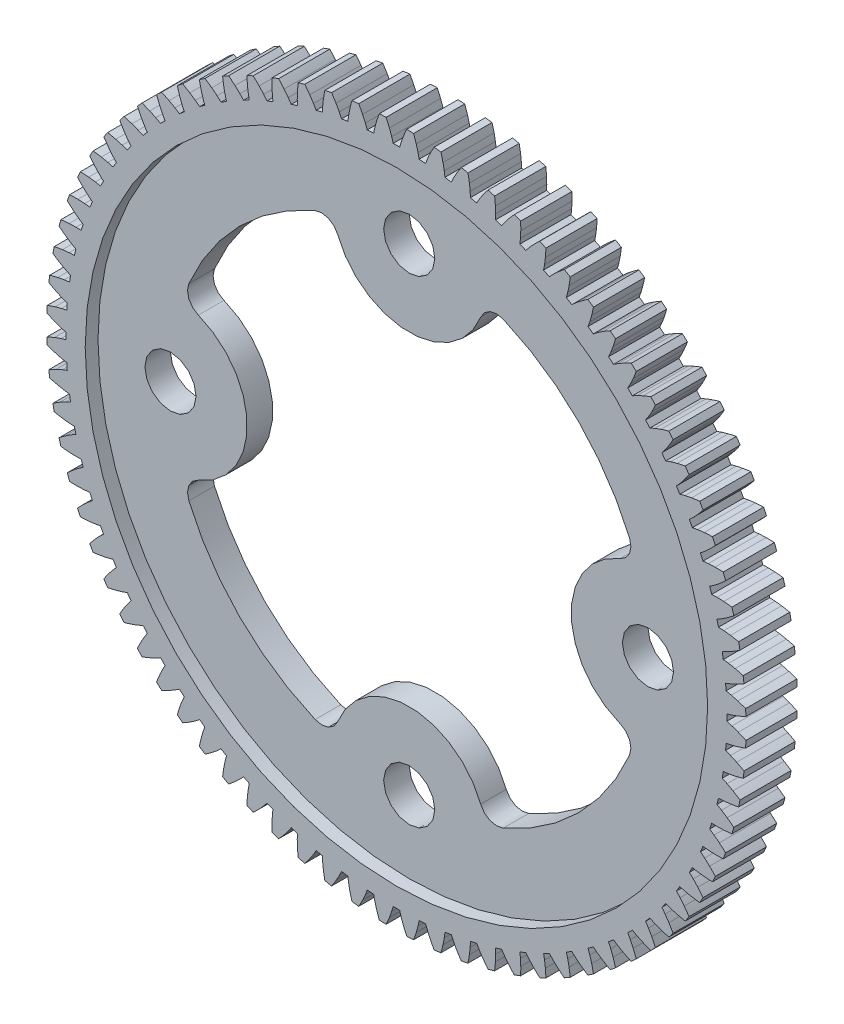
# Autodesk Inventor part: 歯車m0.5.z80
Saved by Autodesk Inventor 2020 (Build 240168000, 168)
## iProperties
Part Number: 歯車m0.5.z80
Material: 鋼、高強度、低合金
Document SubType Name: Modeling
Designer: 雪村
Density: 7.85 g/cm^3
Appearance: 鋼 - つや出し
Mass: 10.9737 g
Surface Area: 25.8897 cm^2
Volume: 1.39793 cm^3
Author: 雪村
Autodesk Inventor part; units mm, degrees
(part 1 of 4)
ref_plane "YZ Plane" through (0, 0, 0) normal (1, 0, 0) x (0, 1, 0)
ref_plane "XZ Plane" through (0, 0, 0) normal (0, 1, 0) x (-1, 0, 0)
ref_plane "XY Plane" through (0, 0, 0) normal (0, 0, 1) x (1, 0, 0)
sketch "スケッチ1" plane through (0, 0, 0) normal (0, 0, 1) x (1, 0, 0)
  arc A0 (1.2215, 23.1029) -> (1.1332, 22.8025) centre (6.2327, 21.4655) ccw
  arc A1 (1.3553, 23.4735) -> (1.2215, 23.1029) centre (7.3125, 21.1133) ccw
  arc A2 (1.5487, 23.9195) -> (1.3553, 23.4735) centre (8.4094, 20.6793) ccw
  arc A3 (-0.323, 23.0641) -> (-0.3875, 22.7577) centre (4.8013, 21.8249) ccw
  arc A4 (-0.2187, 23.444) -> (-0.323, 23.0641) centre (5.9054, 21.5585) ccw
  arc A5 (-0.0608, 23.9038) -> (-0.2187, 23.444) centre (7.0329, 21.2118) ccw
  arc A6 (-1.8597, 22.9042) -> (-1.9, 22.5936) centre (3.346, 22.0709) ccw
  arc A7 (-1.7855, 23.2911) -> (-1.8597, 22.9042) centre (4.4676, 21.8919) ccw
  arc A8 (-1.6642, 23.7619) -> (-1.7855, 23.2911) centre (5.6188, 21.6348) ccw
  arc A9 (-3.3791, 22.6242) -> (-3.3949, 22.3115) centre (1.8759, 22.2019) ccw
  arc A10 (-3.3355, 23.0158) -> (-3.3791, 22.6242) centre (3.0081, 22.1115) ccw
  arc A11 (-3.2515, 23.4946) -> (-3.3355, 23.0158) centre (4.176, 21.9455) ccw
  arc A12 (-4.8718, 22.2259) -> (-4.863, 21.9129) centre (0.4001, 22.2172) ccw
  arc A13 (-4.8591, 22.6197) -> (-4.8718, 22.2259) centre (1.5359, 22.2159) ccw
  arc A14 (-4.813, 23.1036) -> (-4.8591, 22.6197) centre (2.7132, 22.142) ccw
  arc A15 (-6.3287, 21.7117) -> (-6.2954, 21.4003) centre (-1.0724, 22.1166) ccw
  arc A16 (-6.3469, 22.1053) -> (-6.3287, 21.7117) centre (0.06, 22.2045) ccw
  arc A17 (-6.3389, 22.5913) -> (-6.3469, 22.1053) centre (1.2395, 22.2232) ccw
  arc A18 (-7.7408, 21.0848) -> (-7.6832, 20.7769) centre (-2.5324, 21.9009) ccw
  arc A19 (-7.7898, 21.4757) -> (-7.7408, 21.0848) centre (-1.4104, 22.0773) ccw
  arc A20 (-7.82, 21.9609) -> (-7.7898, 21.4757) centre (-0.2361, 22.1885) ccw
  arc A21 (-9.0993, 20.349) -> (-9.0177, 20.0466) centre (-3.971, 21.5712) ccw
  arc A22 (-9.1789, 20.7348) -> (-9.0993, 20.349) centre (-2.8663, 21.8351) ccw
  arc A23 (-9.247, 21.2162) -> (-9.1789, 20.7348) centre (-1.7043, 22.0381) ccw
  arc A24 (-10.3959, 19.5089) -> (-10.2909, 19.2138) centre (-5.3794, 21.1297) ccw
  arc A25 (-10.5055, 19.8873) -> (-10.3959, 19.5089) centre (-4.2988, 21.4794) ccw
  arc A26 (-10.6112, 20.3618) -> (-10.5055, 19.8873) centre (-3.1562, 21.773) ccw
  arc A27 (-11.6226, 18.5696) -> (-11.4947, 18.2837) centre (-6.7487, 20.579) ccw
  arc A28 (-11.7616, 18.9383) -> (-11.6226, 18.5696) centre (-5.6989, 21.0125) ccw
  arc A29 (-11.9041, 19.403) -> (-11.7616, 18.9383) centre (-4.5829, 21.3947) ccw
  arc A30 (-12.7719, 17.537) -> (-12.6219, 17.2621) centre (-8.0706, 19.9226) ccw
  arc A31 (-12.9393, 17.8936) -> (-12.7719, 17.537) centre (-7.058, 20.4371) ccw
  arc A32 (-13.1179, 18.3458) -> (-12.9393, 17.8936) centre (-5.9755, 20.9058) ccw
  arc A33 (-13.8365, 16.4174) -> (-13.6655, 16.1551) centre (-9.3369, 19.1645) ccw
  arc A34 (-14.0314, 16.7598) -> (-13.8365, 16.4174) centre (-8.3678, 19.7569) ccw
  arc A35 (-14.2449, 17.1965) -> (-14.0314, 16.7598) centre (-7.3254, 20.309) ccw
  arc A36 (-14.8101, 15.2177) -> (-14.619, 14.9696) centre (-10.5399, 18.3094) ccw
  arc A37 (-15.0312, 15.5438) -> (-14.8101, 15.2177) centre (-9.6202, 18.976) ccw
  arc A38 (-15.2784, 15.9624) -> (-15.0312, 15.5438) centre (-8.6244, 19.6082) ccw
  arc A39 (-15.6865, 13.9454) -> (-15.4765, 13.713) centre (-11.672, 17.3626) ccw
  arc A40 (-15.9326, 14.2531) -> (-15.6865, 13.9454) centre (-10.8075, 18.0992) ccw
  arc A41 (-16.2118, 14.651) -> (-15.9326, 14.2531) centre (-9.8643, 18.8076) ccw
  arc A42 (-16.4604, 12.6082) -> (-16.2328, 12.393) centre (-12.7264, 16.3298) ccw
  arc A43 (-16.7298, 12.8956) -> (-16.4604, 12.6082) centre (-11.9224, 17.132) ccw
  arc A44 (-17.0394, 13.2704) -> (-16.7298, 12.8956) centre (-11.0376, 17.9123) ccw
  arc A45 (-17.127, 11.2144) -> (-16.8832, 11.0178) centre (-13.6965, 15.2175) ccw
  arc A46 (-17.4181, 11.4798) -> (-17.127, 11.2144) centre (-12.9579, 16.0804) ccw
  arc A47 (-17.7561, 11.8292) -> (-17.4181, 11.4798) centre (-12.1371, 16.9276) ccw
  arc A48 (-17.6821, 9.7726) -> (-17.4237, 9.5957) centre (-14.5763, 14.0325) ccw
  arc A49 (-17.9932, 10.0143) -> (-17.6821, 9.7726) centre (-13.9077, 14.9507) ccw
  arc A50 (-18.3576, 10.3361) -> (-17.9932, 10.0143) centre (-13.1559, 15.8597) ccw
  arc A51 (-18.1225, 8.2917) -> (-17.851, 8.1356) centre (-15.3605, 12.7822) ccw
  arc A52 (-18.4516, 8.5083) -> (-18.1225, 8.2917) centre (-14.7659, 13.7499) ccw
  arc A53 (-18.8401, 8.8005) -> (-18.4516, 8.5083) centre (-14.0878, 14.7151) ccw
  arc A54 (-18.4453, 6.7808) -> (-18.1624, 6.6465) centre (-16.0441, 11.4741) ccw
  arc A55 (-18.7903, 6.9709) -> (-18.4453, 6.7808) centre (-15.5273, 12.4856) ccw
  arc A56 (-19.2006, 7.2317) -> (-18.7903, 6.9709) centre (-14.927, 13.501) ccw
  arc A57 (-18.6485, 5.2492) -> (-18.3559, 5.1375) centre (-16.623, 10.1165) ccw
  arc A58 (-19.0075, 5.4117) -> (-18.6485, 5.2492) centre (-16.1872, 11.1654) ccw
  arc A59 (-19.4369, 5.6395) -> (-19.0075, 5.4117) centre (-15.6684, 12.2248) ccw
  arc A60 (-18.731, 3.7064) -> (-18.4305, 3.6181) centre (-17.0936, 8.7176) ccw
  arc A61 (-19.1016, 3.8402) -> (-18.731, 3.7064) centre (-16.7414, 9.7974) ccw
  arc A62 (-19.5475, 4.0336) -> (-19.1016, 3.8402) centre (-16.3073, 10.8943) ccw
  arc A63 (-18.6921, 2.1619) -> (-18.3857, 2.0974) centre (-17.453, 7.2862) ccw
  arc A64 (-19.0721, 2.2662) -> (-18.6921, 2.1619) centre (-17.1866, 8.3903) ccw
  arc A65 (-19.5319, 2.4241) -> (-19.0721, 2.2662) centre (-16.8399, 9.5178) ccw
  arc A66 (-18.5322, 0.6252) -> (-18.2217, 0.585) centre (-17.6989, 5.8309) ccw
  arc A67 (-18.9192, 0.6994) -> (-18.5322, 0.6252) centre (-17.52, 6.9525) ccw
  arc A68 (-19.3899, 0.8207) -> (-18.9192, 0.6994) centre (-17.2628, 8.1037) ccw
  arc A69 (-18.2523, -0.8942) -> (-17.9395, -0.91) centre (-17.8299, 4.3608) ccw
  arc A70 (-18.6438, -0.8506) -> (-18.2523, -0.8942) centre (-17.7396, 5.493) ccw
  arc A71 (-19.1226, -0.7666) -> (-18.6438, -0.8506) centre (-17.5735, 6.6609) ccw
  arc A72 (-17.8539, -2.3869) -> (-17.5409, -2.3781) centre (-17.8452, 2.885) ccw
  arc A73 (-18.2477, -2.3742) -> (-17.8539, -2.3869) centre (-17.8439, 4.0208) ccw
  arc A74 (-18.7317, -2.3281) -> (-18.2477, -2.3742) centre (-17.7701, 5.1981) ccw
  arc A75 (-17.3397, -3.8438) -> (-17.0283, -3.8105) centre (-17.7447, 1.4125) ccw
  arc A76 (-17.7333, -3.862) -> (-17.3397, -3.8438) centre (-17.8325, 2.5449) ccw
  arc A77 (-18.2193, -3.854) -> (-17.7333, -3.862) centre (-17.8512, 3.7244) ccw
  arc A78 (-16.7128, -5.2559) -> (-16.405, -5.1983) centre (-17.5289, -0.0475) ccw
  arc A79 (-17.1037, -5.3049) -> (-16.7128, -5.2559) centre (-17.7053, 1.0745) ccw
  arc A80 (-17.5889, -5.3351) -> (-17.1037, -5.3049) centre (-17.8165, 2.2488) ccw
  arc A81 (-15.977, -6.6144) -> (-15.6747, -6.5328) centre (-17.1992, -1.4861) ccw
  arc A82 (-16.3629, -6.694) -> (-15.977, -6.6144) centre (-17.4631, -0.3814) ccw
  arc A83 (-16.8442, -6.7621) -> (-16.3629, -6.694) centre (-17.6661, 0.7806) ccw
  arc A84 (-15.1369, -7.911) -> (-14.8419, -7.8059) centre (-16.7577, -2.8945) ccw
  arc A85 (-15.5153, -8.0206) -> (-15.1369, -7.911) centre (-17.1075, -1.8139) ccw
  arc A86 (-15.9898, -8.1263) -> (-15.5153, -8.0206) centre (-17.401, -0.6713) ccw
  arc A87 (-14.1976, -9.1377) -> (-13.9118, -9.0098) centre (-16.2071, -4.2638) ccw
  arc A88 (-14.5663, -9.2767) -> (-14.1976, -9.1377) centre (-16.6405, -3.214) ccw
  arc A89 (-15.0311, -9.4192) -> (-14.5663, -9.2767) centre (-17.0228, -2.098) ccw
  arc A90 (-13.165, -10.287) -> (-12.8901, -10.137) centre (-15.5507, -5.5857) ccw
  arc A91 (-13.5217, -10.4544) -> (-13.165, -10.287) centre (-16.0652, -4.5731) ccw
  arc A92 (-13.9738, -10.633) -> (-13.5217, -10.4544) centre (-16.5338, -3.4906) ccw
  arc A93 (-12.0454, -11.3516) -> (-11.7831, -11.1806) centre (-14.7926, -6.852) ccw
  arc A94 (-12.3878, -11.5465) -> (-12.0454, -11.3516) centre (-15.3849, -5.8829) ccw
  arc A95 (-12.8246, -11.76) -> (-12.3878, -11.5465) centre (-15.9371, -4.8405) ccw
  arc A96 (-10.8458, -12.3252) -> (-10.5977, -12.1341) centre (-13.9375, -8.055) ccw
  arc A97 (-11.1718, -12.5463) -> (-10.8458, -12.3252) centre (-14.604, -7.1353) ccw
  arc A98 (-11.5904, -12.7935) -> (-11.1718, -12.5463) centre (-15.2362, -6.1395) ccw
  arc A99 (-9.5734, -13.2016) -> (-9.3411, -12.9916) centre (-12.9906, -9.1871) ccw
  arc A100 (-9.8811, -13.4476) -> (-9.5734, -13.2016) centre (-13.7273, -8.3226) ccw
  arc A101 (-10.279, -13.7268) -> (-9.8811, -13.4476) centre (-14.4357, -7.3794) ccw
  arc A102 (-8.2362, -13.9755) -> (-8.0211, -13.7479) centre (-11.9579, -10.2415) ccw
  arc A103 (-8.5237, -14.2449) -> (-8.2362, -13.9755) centre (-12.7601, -9.4375) ccw
  arc A104 (-8.8985, -14.5545) -> (-8.5237, -14.2449) centre (-13.5403, -8.5527) ccw
  arc A105 (-6.8424, -14.6421) -> (-6.6458, -14.3983) centre (-10.8456, -11.2116) ccw
  arc A106 (-7.1078, -14.9332) -> (-6.8424, -14.6421) centre (-11.7084, -10.473) ccw
  arc A107 (-7.4572, -15.2712) -> (-7.1078, -14.9332) centre (-12.5556, -9.6522) ccw
  arc A108 (-5.4006, -15.1972) -> (-5.2237, -14.9388) centre (-9.6606, -12.0914) ccw
  arc A109 (-5.6424, -15.5083) -> (-5.4006, -15.1972) centre (-10.5787, -11.4228) ccw
  arc A110 (-5.9641, -15.8727) -> (-5.6424, -15.5083) centre (-11.4877, -10.671) ccw
  arc A111 (-3.9197, -15.6376) -> (-3.7636, -15.3661) centre (-8.4102, -12.8756) ccw
  arc A112 (-4.1363, -15.9667) -> (-3.9197, -15.6376) centre (-9.378, -12.281) ccw
  arc A113 (-4.4285, -16.3552) -> (-4.1363, -15.9667) centre (-10.3432, -11.6029) ccw
  arc A114 (-2.4088, -15.9604) -> (-2.2745, -15.6774) centre (-7.1022, -13.5592) ccw
  arc A115 (-2.5989, -16.3054) -> (-2.4088, -15.9604) centre (-8.1136, -13.0424) ccw
  arc A116 (-2.8597, -16.7157) -> (-2.5989, -16.3054) centre (-9.129, -12.4421) ccw
  arc A117 (-0.8773, -16.1636) -> (-0.7656, -15.871) centre (-5.7445, -14.1381) ccw
  arc A118 (-1.0397, -16.5225) -> (-0.8773, -16.1636) centre (-6.7934, -13.7022) ccw
  arc A119 (-1.2675, -16.952) -> (-1.0397, -16.5225) centre (-7.8528, -13.1834) ccw
  arc A120 (0.6655, -16.2461) -> (0.7539, -15.9456) centre (-4.3457, -14.6087) ccw
  arc A121 (0.5317, -16.6166) -> (0.6655, -16.2461) centre (-5.4255, -14.2565) ccw
  arc A122 (0.3383, -17.0626) -> (0.5317, -16.6166) centre (-6.5223, -13.8224) ccw
  arc A123 (2.21, -16.2072) -> (2.2746, -15.9008) centre (-2.9142, -14.9681) ccw
  arc A124 (2.1057, -16.5872) -> (2.21, -16.2072) centre (-4.0183, -14.7017) ccw
  arc A125 (1.9479, -17.0469) -> (2.1057, -16.5872) centre (-5.1458, -14.355) ccw
  arc A126 (3.7467, -16.0473) -> (3.787, -15.7368) centre (-1.4589, -15.214) ccw
  arc A127 (3.6725, -16.4343) -> (3.7467, -16.0473) centre (-2.5805, -15.0351) ccw
  arc A128 (3.5513, -16.905) -> (3.6725, -16.4343) centre (-3.7318, -14.7779) ccw
  arc A129 (5.2661, -15.7674) -> (5.2819, -15.4546) centre (0.0111, -15.345) ccw
  arc A130 (5.2225, -16.1589) -> (5.2661, -15.7674) centre (-1.121, -15.2547) ccw
  arc A131 (5.1386, -16.6377) -> (5.2225, -16.1589) centre (-2.2889, -15.0886) ccw
  arc A132 (6.7589, -15.369) -> (6.7501, -15.056) centre (1.487, -15.3603) ccw
  arc A133 (6.7462, -15.7628) -> (6.7589, -15.369) centre (0.3512, -15.359) ccw
  arc A134 (6.7, -16.2467) -> (6.7462, -15.7628) centre (-0.8261, -15.2851) ccw
  arc A135 (8.2158, -14.8548) -> (8.1825, -14.5434) centre (2.9594, -15.2598) ccw
  arc A136 (8.234, -15.2484) -> (8.2158, -14.8548) centre (1.827, -15.3476) ccw
  arc A137 (8.226, -15.7344) -> (8.234, -15.2484) centre (0.6476, -15.3663) ccw
  arc A138 (9.6279, -14.2279) -> (9.5702, -13.9201) centre (4.4195, -15.044) ccw
  arc A139 (9.6769, -14.6188) -> (9.6279, -14.2279) centre (3.2975, -15.2204) ccw
  arc A140 (9.707, -15.104) -> (9.6769, -14.6188) centre (2.1231, -15.3316) ccw
  arc A141 (10.9864, -13.4921) -> (10.9048, -13.1898) centre (5.8581, -14.7143) ccw
  arc A142 (11.0659, -13.878) -> (10.9864, -13.4921) centre (4.7534, -14.9782) ccw
  arc A143 (11.1341, -14.3593) -> (11.0659, -13.878) centre (3.5914, -15.1812) ccw
  arc A144 (12.283, -12.652) -> (12.1779, -12.357) centre (7.2664, -14.2728) ccw
  arc A145 (12.3926, -13.0304) -> (12.283, -12.652) centre (6.1858, -14.6226) ccw
  arc A146 (12.4983, -13.5049) -> (12.3926, -13.0304) centre (5.0433, -14.9161) ccw
  arc A147 (13.5097, -11.7127) -> (13.3818, -11.4269) centre (8.6357, -13.7222) ccw
  arc A148 (13.6486, -12.0814) -> (13.5097, -11.7127) centre (7.5859, -14.1556) ccw
  arc A149 (13.7912, -12.5461) -> (13.6486, -12.0814) centre (6.47, -14.5379) ccw
  arc A150 (14.6589, -10.6801) -> (14.509, -10.4052) centre (9.9577, -13.0658) ccw
  arc A151 (14.8264, -11.0368) -> (14.6589, -10.6801) centre (8.9451, -13.5803) ccw
  arc A152 (15.005, -11.4889) -> (14.8264, -11.0368) centre (7.8625, -14.0489) ccw
  arc A153 (15.7236, -9.5605) -> (15.5525, -9.2982) centre (11.224, -12.3077) ccw
  arc A154 (15.9185, -9.9029) -> (15.7236, -9.5605) centre (10.2549, -12.9) ccw
  arc A155 (16.132, -10.3397) -> (15.9185, -9.9029) centre (9.2125, -13.4522) ccw
  arc A156 (16.6971, -8.3609) -> (16.506, -8.1128) centre (12.4269, -11.4526) ccw
  arc A157 (16.9183, -8.6869) -> (16.6971, -8.3609) centre (11.5073, -12.1191) ccw
  arc A158 (17.1654, -9.1055) -> (16.9183, -8.6869) centre (10.5114, -12.7513) ccw
  arc A159 (17.5735, -7.0885) -> (17.3636, -6.8562) centre (13.5591, -10.5057) ccw
  arc A160 (17.8196, -7.3962) -> (17.5735, -7.0885) centre (12.6946, -11.2424) ccw
  arc A161 (18.0988, -7.7941) -> (17.8196, -7.3962) centre (11.7514, -11.9508) ccw
  arc A162 (18.3474, -5.7513) -> (18.1199, -5.5362) centre (14.6135, -9.473) ccw
  arc A163 (18.6169, -6.0388) -> (18.3474, -5.7513) centre (13.8094, -10.2752) ccw
  arc A164 (18.9264, -6.4136) -> (18.6169, -6.0388) centre (12.9247, -11.0554) ccw
  arc A165 (19.014, -4.3575) -> (18.7703, -4.1609) centre (15.5835, -8.3607) ccw
  arc A166 (19.3052, -4.6229) -> (19.014, -4.3575) centre (14.8449, -9.2235) ccw
  arc A167 (19.6432, -4.9723) -> (19.3052, -4.6229) centre (14.0242, -10.0707) ccw
  arc A168 (19.5692, -2.9157) -> (19.3108, -2.7388) centre (16.4634, -7.1757) ccw
  arc A169 (19.8803, -3.1575) -> (19.5692, -2.9157) centre (15.7947, -8.0938) ccw
  arc A170 (20.2447, -3.4792) -> (19.8803, -3.1575) centre (15.043, -9.0028) ccw
  arc A171 (20.0095, -1.4348) -> (19.738, -1.2787) centre (17.2475, -5.9253) ccw
  arc A172 (20.3386, -1.6514) -> (20.0095, -1.4348) centre (16.653, -6.8931) ccw
  arc A173 (20.7271, -1.9436) -> (20.3386, -1.6514) centre (15.9748, -7.8583) ccw
  arc A174 (20.3323, 0.0761) -> (20.0494, 0.2104) centre (17.9312, -4.6173) ccw
  arc A175 (20.6774, -0.114) -> (20.3323, 0.0761) centre (17.4144, -5.6287) ccw
  arc A176 (21.0876, -0.3748) -> (20.6774, -0.114) centre (16.814, -6.6441) ccw
  arc A177 (20.5356, 1.6076) -> (20.243, 1.7193) centre (18.51, -3.2596) ccw
  arc A178 (20.8945, 1.4452) -> (20.5356, 1.6076) centre (18.0742, -4.3085) ccw
  arc A179 (21.3239, 1.2174) -> (20.8945, 1.4452) centre (17.5554, -5.3679) ccw
  arc A180 (20.618, 3.1504) -> (20.3176, 3.2388) centre (18.9806, -1.8608) ccw
  arc A181 (20.9886, 3.0166) -> (20.618, 3.1504) centre (18.6284, -2.9406) ccw
  arc A182 (21.4346, 2.8232) -> (20.9886, 3.0166) centre (18.1944, -4.0374) ccw
  arc A183 (20.5792, 4.6949) -> (20.2728, 4.7595) centre (19.34, -0.4293) ccw
  arc A184 (20.9591, 4.5906) -> (20.5792, 4.6949) centre (19.0736, -1.5334) ccw
  arc A185 (21.4189, 4.4328) -> (20.9591, 4.5906) centre (18.7269, -2.6609) ccw
  arc A186 (20.4193, 6.2316) -> (20.1087, 6.2719) centre (19.586, 1.026) ccw
  arc A187 (20.8062, 6.1575) -> (20.4193, 6.2316) centre (19.407, -0.0956) ccw
  arc A188 (21.277, 6.0362) -> (20.8062, 6.1575) centre (19.1499, -1.2469) ccw
  arc A189 (20.1393, 7.751) -> (19.8266, 7.7668) centre (19.717, 2.496) ccw
  arc A190 (20.5309, 7.7074) -> (20.1393, 7.751) centre (19.6266, 1.3639) ccw
  arc A191 (21.0097, 7.6235) -> (20.5309, 7.7074) centre (19.4606, 0.196) ccw
  arc A192 (19.741, 9.2438) -> (19.428, 9.235) centre (19.7323, 3.9719) ccw
  arc A193 (20.1348, 9.2311) -> (19.741, 9.2438) centre (19.731, 2.8361) ccw
  arc A194 (20.6187, 9.1849) -> (20.1348, 9.2311) centre (19.6571, 1.6588) ccw
  arc A195 (19.2268, 10.7007) -> (18.9154, 10.6674) centre (19.6317, 5.4443) ccw
  arc A196 (19.6204, 10.7189) -> (19.2268, 10.7007) centre (19.7196, 4.312) ccw
  arc A197 (20.1064, 10.7109) -> (19.6204, 10.7189) centre (19.7383, 3.1325) ccw
  arc A198 (18.5999, 12.1128) -> (18.292, 12.0551) centre (19.416, 6.9044) ccw
  arc A199 (18.9908, 12.1618) -> (18.5999, 12.1128) centre (19.5924, 5.7824) ccw
  arc A200 (19.476, 12.1919) -> (18.9908, 12.1618) centre (19.7035, 4.608) ccw
  arc A201 (17.8641, 13.4713) -> (17.5617, 13.3897) centre (19.0863, 8.343) ccw
  arc A202 (18.2499, 13.5508) -> (17.8641, 13.4713) centre (19.3502, 7.2383) ccw
  arc A203 (18.7313, 13.619) -> (18.2499, 13.5508) centre (19.5532, 6.0763) ccw
  arc A204 (17.024, 14.7679) -> (16.7289, 14.6628) centre (18.6448, 9.7513) ccw
  arc A205 (17.4024, 14.8775) -> (17.024, 14.7679) centre (18.9945, 8.6707) ccw
  arc A206 (17.8769, 14.9832) -> (17.4024, 14.8775) centre (19.2881, 7.5282) ccw
  arc A207 (16.0847, 15.9946) -> (15.7988, 15.8667) centre (18.0941, 11.1207) ccw
  arc A208 (16.4534, 16.1335) -> (16.0847, 15.9946) centre (18.5276, 10.0708) ccw
  arc A209 (16.9181, 16.2761) -> (16.4534, 16.1335) centre (18.9098, 8.9549) ccw
  arc A210 (15.0521, 17.1438) -> (14.7772, 16.9939) centre (17.4377, 12.4426) ccw
  arc A211 (15.4087, 17.3113) -> (15.0521, 17.1438) centre (17.9522, 11.43) ccw
  arc A212 (15.8608, 17.4899) -> (15.4087, 17.3113) centre (18.4209, 10.3475) ccw
  arc A213 (13.9325, 18.2085) -> (13.6702, 18.0374) centre (16.6796, 13.7089) ccw
  arc A214 (14.2749, 18.4034) -> (13.9325, 18.2085) centre (17.272, 12.7398) ccw
  arc A215 (14.7116, 18.6169) -> (14.2749, 18.4034) centre (17.8241, 11.6974) ccw
  arc A216 (12.7328, 19.182) -> (12.4847, 18.9909) centre (15.8245, 14.9118) ccw
  arc A217 (13.0589, 19.4032) -> (12.7328, 19.182) centre (16.4911, 13.9922) ccw
  arc A218 (13.4775, 19.6503) -> (13.0589, 19.4032) centre (17.1233, 12.9963) ccw
  arc A219 (11.4605, 20.0585) -> (11.2281, 19.8485) centre (14.8777, 16.044) ccw
  arc A220 (11.7682, 20.3045) -> (11.4605, 20.0585) centre (15.6143, 15.1795) ccw
  arc A221 (12.1661, 20.5837) -> (11.7682, 20.3045) centre (16.3227, 14.2363) ccw
  arc A222 (10.1233, 20.8323) -> (9.9081, 20.6048) centre (13.8449, 17.0984) ccw
  arc A223 (10.4107, 21.1018) -> (10.1233, 20.8323) centre (14.6471, 16.2943) ccw
  arc A224 (10.7855, 21.4113) -> (10.4107, 21.1018) centre (15.4274, 15.4096) ccw
  arc A225 (8.7295, 21.4989) -> (8.5329, 21.2552) centre (12.7326, 18.0685) ccw
  arc A226 (8.9949, 21.7901) -> (8.7295, 21.4989) centre (13.5955, 17.3298) ccw
  arc A227 (9.3443, 22.1281) -> (8.9949, 21.7901) centre (14.4427, 16.5091) ccw
  arc A228 (7.2877, 22.0541) -> (7.1108, 21.7957) centre (11.5476, 18.9483) ccw
  arc A229 (7.5294, 22.3652) -> (7.2877, 22.0541) centre (12.4658, 18.2796) ccw
  arc A230 (7.8512, 22.7296) -> (7.5294, 22.3652) centre (13.3748, 17.5279) ccw
  arc A231 (5.8068, 22.4944) -> (5.6507, 22.2229) centre (10.2973, 19.7324) ccw
  arc A232 (6.0234, 22.8235) -> (5.8068, 22.4944) centre (11.265, 19.1379) ccw
  arc A233 (6.3156, 23.212) -> (6.0234, 22.8235) centre (12.2302, 18.4597) ccw
  arc A234 (4.2959, 22.8172) -> (4.1616, 22.5343) centre (8.9892, 20.4161) ccw
  arc A235 (4.486, 23.1623) -> (4.2959, 22.8172) centre (10.0007, 19.8993) ccw
  arc A236 (4.7468, 23.5725) -> (4.486, 23.1623) centre (11.0161, 19.299) ccw
  arc A237 (2.7643, 23.0205) -> (2.6526, 22.7279) centre (7.6316, 20.995) ccw
  arc A238 (2.9268, 23.3794) -> (2.7643, 23.0205) centre (8.6805, 20.5591) ccw
  arc A239 (3.1546, 23.8088) -> (2.9268, 23.3794) centre (9.7398, 20.0403) ccw
  arc A240 (0.7539, 22.8025) -> (0.6655, 23.1029) centre (-4.3457, 21.4655) ccw
  arc A241 (0.6655, 23.1029) -> (0.5317, 23.4735) centre (-5.4255, 21.1133) ccw
  arc A242 (0.5317, 23.4735) -> (0.3383, 23.9195) centre (-6.5223, 20.6793) ccw
  arc A243 (-0.7656, 22.7279) -> (-0.8773, 23.0205) centre (-5.7445, 20.995) ccw
  arc A244 (-0.8773, 23.0205) -> (-1.0397, 23.3794) centre (-6.7934, 20.5591) ccw
  arc A245 (-1.0397, 23.3794) -> (-1.2675, 23.8088) centre (-7.8528, 20.0403) ccw
  arc A246 (-2.2745, 22.5343) -> (-2.4088, 22.8172) centre (-7.1022, 20.4161) ccw
  arc A247 (-2.4088, 22.8172) -> (-2.5989, 23.1623) centre (-8.1136, 19.8993) ccw
  arc A248 (-2.5989, 23.1623) -> (-2.8597, 23.5725) centre (-9.129, 19.299) ccw
  arc A249 (-3.7636, 22.2229) -> (-3.9197, 22.4944) centre (-8.4102, 19.7324) ccw
  arc A250 (-3.9197, 22.4944) -> (-4.1363, 22.8235) centre (-9.378, 19.1379) ccw
  arc A251 (-4.1363, 22.8235) -> (-4.4285, 23.212) centre (-10.3432, 18.4597) ccw
  arc A252 (-5.2237, 21.7957) -> (-5.4006, 22.0541) centre (-9.6606, 18.9483) ccw
  arc A253 (-5.4006, 22.0541) -> (-5.6424, 22.3652) centre (-10.5787, 18.2796) ccw
  arc A254 (-5.6424, 22.3652) -> (-5.9641, 22.7296) centre (-11.4877, 17.5279) ccw
  arc A255 (-6.6458, 21.2552) -> (-6.8424, 21.4989) centre (-10.8456, 18.0685) ccw
  arc A256 (-6.8424, 21.4989) -> (-7.1078, 21.7901) centre (-11.7084, 17.3298) ccw
  arc A257 (-7.1078, 21.7901) -> (-7.4572, 22.1281) centre (-12.5556, 16.5091) ccw
  arc A258 (-8.0211, 20.6048) -> (-8.2362, 20.8323) centre (-11.9579, 17.0984) ccw
  arc A259 (-8.2362, 20.8323) -> (-8.5237, 21.1018) centre (-12.7601, 16.2943) ccw
  arc A260 (-8.5237, 21.1018) -> (-8.8985, 21.4113) centre (-13.5403, 15.4096) ccw
  arc A261 (-9.3411, 19.8485) -> (-9.5734, 20.0585) centre (-12.9906, 16.044) ccw
  arc A262 (-9.5734, 20.0585) -> (-9.8811, 20.3045) centre (-13.7273, 15.1795) ccw
  arc A263 (-9.8811, 20.3045) -> (-10.279, 20.5837) centre (-14.4357, 14.2363) ccw
  arc A264 (-10.5977, 18.9909) -> (-10.8458, 19.182) centre (-13.9375, 14.9118) ccw
  arc A265 (-10.8458, 19.182) -> (-11.1718, 19.4032) centre (-14.604, 13.9922) ccw
  arc A266 (-11.1718, 19.4032) -> (-11.5904, 19.6503) centre (-15.2362, 12.9963) ccw
  arc A267 (-11.7831, 18.0374) -> (-12.0454, 18.2085) centre (-14.7926, 13.7089) ccw
  arc A268 (-12.0454, 18.2085) -> (-12.3878, 18.4034) centre (-15.3849, 12.7398) ccw
  arc A269 (-12.3878, 18.4034) -> (-12.8246, 18.6169) centre (-15.9371, 11.6974) ccw
  arc A270 (-12.8901, 16.9939) -> (-13.165, 17.1438) centre (-15.5507, 12.4426) ccw
  arc A271 (-13.165, 17.1438) -> (-13.5217, 17.3113) centre (-16.0652, 11.43) ccw
  arc A272 (-13.5217, 17.3113) -> (-13.9738, 17.4899) centre (-16.5338, 10.3475) ccw
  arc A273 (-13.9118, 15.8667) -> (-14.1976, 15.9946) centre (-16.2071, 11.1207) ccw
  arc A274 (-14.1976, 15.9946) -> (-14.5663, 16.1335) centre (-16.6405, 10.0708) ccw
  arc A275 (-14.5663, 16.1335) -> (-15.0311, 16.2761) centre (-17.0228, 8.9549) ccw
  arc A276 (-14.8419, 14.6628) -> (-15.1369, 14.7679) centre (-16.7577, 9.7513) ccw
  arc A277 (-15.1369, 14.7679) -> (-15.5153, 14.8775) centre (-17.1075, 8.6707) ccw
  arc A278 (-15.5153, 14.8775) -> (-15.9898, 14.9832) centre (-17.401, 7.5282) ccw
  arc A279 (-15.6747, 13.3897) -> (-15.977, 13.4713) centre (-17.1992, 8.343) ccw
  arc A280 (-15.977, 13.4713) -> (-16.3629, 13.5508) centre (-17.4631, 7.2383) ccw
  arc A281 (-16.3629, 13.5508) -> (-16.8442, 13.619) centre (-17.6661, 6.0763) ccw
  arc A282 (-16.405, 12.0551) -> (-16.7128, 12.1128) centre (-17.5289, 6.9044) ccw
  arc A283 (-16.7128, 12.1128) -> (-17.1037, 12.1618) centre (-17.7053, 5.7824) ccw
  arc A284 (-17.1037, 12.1618) -> (-17.5889, 12.1919) centre (-17.8165, 4.608) ccw
  arc A285 (-17.0283, 10.6674) -> (-17.3397, 10.7007) centre (-17.7447, 5.4443) ccw
  arc A286 (-17.3397, 10.7007) -> (-17.7333, 10.7189) centre (-17.8325, 4.312) ccw
  arc A287 (-17.7333, 10.7189) -> (-18.2193, 10.7109) centre (-17.8512, 3.1325) ccw
  arc A288 (-17.5409, 9.235) -> (-17.8539, 9.2438) centre (-17.8452, 3.9719) ccw
  arc A289 (-17.8539, 9.2438) -> (-18.2477, 9.2311) centre (-17.8439, 2.8361) ccw
  arc A290 (-18.2477, 9.2311) -> (-18.7317, 9.1849) centre (-17.7701, 1.6588) ccw
  arc A291 (-17.9395, 7.7668) -> (-18.2523, 7.751) centre (-17.8299, 2.496) ccw
  arc A292 (-18.2523, 7.751) -> (-18.6438, 7.7074) centre (-17.7396, 1.3639) ccw
  arc A293 (-18.6438, 7.7074) -> (-19.1226, 7.6235) centre (-17.5735, 0.196) ccw
  arc A294 (-18.2217, 6.2719) -> (-18.5322, 6.2316) centre (-17.6989, 1.026) ccw
  arc A295 (-18.5322, 6.2316) -> (-18.9192, 6.1575) centre (-17.52, -0.0956) ccw
  arc A296 (-18.9192, 6.1575) -> (-19.3899, 6.0362) centre (-17.2628, -1.2469) ccw
  arc A297 (-18.3857, 4.7595) -> (-18.6921, 4.6949) centre (-17.453, -0.4293) ccw
  arc A298 (-18.6921, 4.6949) -> (-19.0721, 4.5906) centre (-17.1866, -1.5334) ccw
  arc A299 (-19.0721, 4.5906) -> (-19.5319, 4.4328) centre (-16.8399, -2.6609) ccw
  arc A300 (-18.4305, 3.2388) -> (-18.731, 3.1504) centre (-17.0936, -1.8608) ccw
  arc A301 (-18.731, 3.1504) -> (-19.1016, 3.0166) centre (-16.7414, -2.9406) ccw
  arc A302 (-19.1016, 3.0166) -> (-19.5475, 2.8232) centre (-16.3073, -4.0374) ccw
  arc A303 (-18.3559, 1.7193) -> (-18.6485, 1.6076) centre (-16.623, -3.2596) ccw
  arc A304 (-18.6485, 1.6076) -> (-19.0075, 1.4452) centre (-16.1872, -4.3085) ccw
  arc A305 (-19.0075, 1.4452) -> (-19.4369, 1.2174) centre (-15.6684, -5.3679) ccw
  arc A306 (-18.1624, 0.2104) -> (-18.4453, 0.0761) centre (-16.0441, -4.6173) ccw
  arc A307 (-18.4453, 0.0761) -> (-18.7903, -0.114) centre (-15.5273, -5.6287) ccw
  arc A308 (-18.7903, -0.114) -> (-19.2006, -0.3748) centre (-14.927, -6.6441) ccw
  arc A309 (-17.851, -1.2787) -> (-18.1225, -1.4348) centre (-15.3605, -5.9253) ccw
  arc A310 (-18.1225, -1.4348) -> (-18.4516, -1.6514) centre (-14.7659, -6.8931) ccw
  arc A311 (-18.4516, -1.6514) -> (-18.8401, -1.9436) centre (-14.0878, -7.8583) ccw
  arc A312 (-17.4237, -2.7388) -> (-17.6821, -2.9157) centre (-14.5763, -7.1757) ccw
  arc A313 (-17.6821, -2.9157) -> (-17.9932, -3.1575) centre (-13.9077, -8.0938) ccw
  arc A314 (-17.9932, -3.1575) -> (-18.3576, -3.4792) centre (-13.1559, -9.0028) ccw
  arc A315 (-16.8832, -4.1609) -> (-17.127, -4.3575) centre (-13.6965, -8.3607) ccw
  arc A316 (-17.127, -4.3575) -> (-17.4181, -4.6229) centre (-12.9579, -9.2235) ccw
  arc A317 (-17.4181, -4.6229) -> (-17.7561, -4.9723) centre (-12.1371, -10.0707) ccw
  arc A318 (-16.2328, -5.5362) -> (-16.4604, -5.7513) centre (-12.7264, -9.473) ccw
  arc A319 (-16.4604, -5.7513) -> (-16.7298, -6.0388) centre (-11.9224, -10.2752) ccw
  arc A320 (-16.7298, -6.0388) -> (-17.0394, -6.4136) centre (-11.0376, -11.0554) ccw
  arc A321 (-15.4765, -6.8562) -> (-15.6865, -7.0885) centre (-11.672, -10.5057) ccw
  arc A322 (-15.6865, -7.0885) -> (-15.9326, -7.3962) centre (-10.8075, -11.2424) ccw
  arc A323 (-15.9326, -7.3962) -> (-16.2118, -7.7941) centre (-9.8643, -11.9508) ccw
  arc A324 (-14.619, -8.1128) -> (-14.8101, -8.3609) centre (-10.5399, -11.4526) ccw
  arc A325 (-14.8101, -8.3609) -> (-15.0312, -8.6869) centre (-9.6202, -12.1191) ccw
  arc A326 (-15.0312, -8.6869) -> (-15.2784, -9.1055) centre (-8.6244, -12.7513) ccw
  arc A327 (-13.6655, -9.2982) -> (-13.8365, -9.5605) centre (-9.3369, -12.3077) ccw
  arc A328 (-13.8365, -9.5605) -> (-14.0314, -9.9029) centre (-8.3678, -12.9) ccw
  arc A329 (-14.0314, -9.9029) -> (-14.2449, -10.3397) centre (-7.3254, -13.4522) ccw
  arc A330 (-12.6219, -10.4052) -> (-12.7719, -10.6801) centre (-8.0706, -13.0658) ccw
  arc A331 (-12.7719, -10.6801) -> (-12.9393, -11.0368) centre (-7.058, -13.5803) ccw
  arc A332 (-12.9393, -11.0368) -> (-13.1179, -11.4889) centre (-5.9755, -14.0489) ccw
  arc A333 (-11.4947, -11.4269) -> (-11.6226, -11.7127) centre (-6.7487, -13.7222) ccw
  arc A334 (-11.6226, -11.7127) -> (-11.7616, -12.0814) centre (-5.6989, -14.1556) ccw
  arc A335 (-11.7616, -12.0814) -> (-11.9041, -12.5461) centre (-4.5829, -14.5379) ccw
  arc A336 (-10.2909, -12.357) -> (-10.3959, -12.652) centre (-5.3794, -14.2728) ccw
  arc A337 (-10.3959, -12.652) -> (-10.5055, -13.0304) centre (-4.2988, -14.6226) ccw
  arc A338 (-10.5055, -13.0304) -> (-10.6112, -13.5049) centre (-3.1562, -14.9161) ccw
  arc A339 (-9.0177, -13.1898) -> (-9.0993, -13.4921) centre (-3.971, -14.7143) ccw
  arc A340 (-9.0993, -13.4921) -> (-9.1789, -13.878) centre (-2.8663, -14.9782) ccw
  arc A341 (-9.1789, -13.878) -> (-9.247, -14.3593) centre (-1.7043, -15.1812) ccw
  arc A342 (-7.6832, -13.9201) -> (-7.7408, -14.2279) centre (-2.5324, -15.044) ccw
  arc A343 (-7.7408, -14.2279) -> (-7.7898, -14.6188) centre (-1.4104, -15.2204) ccw
  arc A344 (-7.7898, -14.6188) -> (-7.82, -15.104) centre (-0.2361, -15.3316) ccw
  arc A345 (-6.2954, -14.5434) -> (-6.3287, -14.8548) centre (-1.0724, -15.2598) ccw
  arc A346 (-6.3287, -14.8548) -> (-6.3469, -15.2484) centre (0.06, -15.3476) ccw
  arc A347 (-6.3469, -15.2484) -> (-6.3389, -15.7344) centre (1.2395, -15.3663) ccw
  arc A348 (-4.863, -15.056) -> (-4.8718, -15.369) centre (0.4001, -15.3603) ccw
  arc A349 (-4.8718, -15.369) -> (-4.8591, -15.7628) centre (1.5359, -15.359) ccw
  arc A350 (-4.8591, -15.7628) -> (-4.813, -16.2467) centre (2.7132, -15.2851) ccw
  arc A351 (-3.3949, -15.4546) -> (-3.3791, -15.7674) centre (1.8759, -15.345) ccw
  arc A352 (-3.3791, -15.7674) -> (-3.3355, -16.1589) centre (3.0081, -15.2547) ccw
  arc A353 (-3.3355, -16.1589) -> (-3.2515, -16.6377) centre (4.176, -15.0886) ccw
  arc A354 (-1.9, -15.7368) -> (-1.8597, -16.0473) centre (3.346, -15.214) ccw
  arc A355 (-1.8597, -16.0473) -> (-1.7855, -16.4343) centre (4.4676, -15.0351) ccw
  arc A356 (-1.7855, -16.4343) -> (-1.6642, -16.905) centre (5.6188, -14.7779) ccw
  arc A357 (-0.3875, -15.9008) -> (-0.323, -16.2072) centre (4.8013, -14.9681) ccw
  arc A358 (-0.323, -16.2072) -> (-0.2187, -16.5872) centre (5.9054, -14.7017) ccw
  arc A359 (-0.2187, -16.5872) -> (-0.0608, -17.0469) centre (7.0329, -14.355) ccw
  arc A360 (1.1332, -15.9456) -> (1.2215, -16.2461) centre (6.2327, -14.6087) ccw
  arc A361 (1.2215, -16.2461) -> (1.3553, -16.6166) centre (7.3125, -14.2565) ccw
  arc A362 (1.3553, -16.6166) -> (1.5487, -17.0626) centre (8.4094, -13.8224) ccw
  arc A363 (2.6526, -15.871) -> (2.7643, -16.1636) centre (7.6316, -14.1381) ccw
  arc A364 (2.7643, -16.1636) -> (2.9268, -16.5225) centre (8.6805, -13.7022) ccw
  arc A365 (2.9268, -16.5225) -> (3.1546, -16.952) centre (9.7398, -13.1834) ccw
  arc A366 (4.1616, -15.6774) -> (4.2959, -15.9604) centre (8.9892, -13.5592) ccw
  arc A367 (4.2959, -15.9604) -> (4.486, -16.3054) centre (10.0007, -13.0424) ccw
  arc A368 (4.486, -16.3054) -> (4.7468, -16.7157) centre (11.0161, -12.4421) ccw
  arc A369 (5.6507, -15.3661) -> (5.8068, -15.6376) centre (10.2973, -12.8756) ccw
  arc A370 (5.8068, -15.6376) -> (6.0234, -15.9667) centre (11.265, -12.281) ccw
  arc A371 (6.0234, -15.9667) -> (6.3156, -16.3552) centre (12.2302, -11.6029) ccw
  arc A372 (7.1108, -14.9388) -> (7.2877, -15.1972) centre (11.5476, -12.0914) ccw
  arc A373 (7.2877, -15.1972) -> (7.5294, -15.5083) centre (12.4658, -11.4228) ccw
  arc A374 (7.5294, -15.5083) -> (7.8512, -15.8727) centre (13.3748, -10.671) ccw
  arc A375 (8.5329, -14.3983) -> (8.7295, -14.6421) centre (12.7326, -11.2116) ccw
  arc A376 (8.7295, -14.6421) -> (8.9949, -14.9332) centre (13.5955, -10.473) ccw
  arc A377 (8.9949, -14.9332) -> (9.3443, -15.2712) centre (14.4427, -9.6522) ccw
  arc A378 (9.9081, -13.7479) -> (10.1233, -13.9755) centre (13.8449, -10.2415) ccw
  arc A379 (10.1233, -13.9755) -> (10.4107, -14.2449) centre (14.6471, -9.4375) ccw
  arc A380 (10.4107, -14.2449) -> (10.7855, -14.5545) centre (15.4274, -8.5527) ccw
  arc A381 (11.2281, -12.9916) -> (11.4605, -13.2016) centre (14.8777, -9.1871) ccw
  arc A382 (11.4605, -13.2016) -> (11.7682, -13.4476) centre (15.6143, -8.3226) ccw
  arc A383 (11.7682, -13.4476) -> (12.1661, -13.7268) centre (16.3227, -7.3794) ccw
  arc A384 (12.4847, -12.1341) -> (12.7328, -12.3252) centre (15.8245, -8.055) ccw
  arc A385 (12.7328, -12.3252) -> (13.0589, -12.5463) centre (16.4911, -7.1353) ccw
  arc A386 (13.0589, -12.5463) -> (13.4775, -12.7935) centre (17.1233, -6.1395) ccw
  arc A387 (13.6702, -11.1806) -> (13.9325, -11.3516) centre (16.6796, -6.852) ccw
  arc A388 (13.9325, -11.3516) -> (14.2749, -11.5465) centre (17.272, -5.8829) ccw
  arc A389 (14.2749, -11.5465) -> (14.7116, -11.76) centre (17.8241, -4.8405) ccw
  arc A390 (14.7772, -10.137) -> (15.0521, -10.287) centre (17.4377, -5.5857) ccw
  arc A391 (15.0521, -10.287) -> (15.4087, -10.4544) centre (17.9522, -4.5731) ccw
  arc A392 (15.4087, -10.4544) -> (15.8608, -10.633) centre (18.4209, -3.4906) ccw
  arc A393 (15.7988, -9.0098) -> (16.0847, -9.1377) centre (18.0941, -4.2638) ccw
  arc A394 (16.0847, -9.1377) -> (16.4534, -9.2767) centre (18.5276, -3.214) ccw
  arc A395 (16.4534, -9.2767) -> (16.9181, -9.4192) centre (18.9098, -2.098) ccw
  arc A396 (16.7289, -7.8059) -> (17.024, -7.911) centre (18.6448, -2.8945) ccw
  arc A397 (17.024, -7.911) -> (17.4024, -8.0206) centre (18.9945, -1.8139) ccw
  arc A398 (17.4024, -8.0206) -> (17.8769, -8.1263) centre (19.2881, -0.6713) ccw
  arc A399 (17.5617, -6.5328) -> (17.8641, -6.6144) centre (19.0863, -1.4861) ccw
  arc A400 (17.8641, -6.6144) -> (18.2499, -6.694) centre (19.3502, -0.3814) ccw
  arc A401 (18.2499, -6.694) -> (18.7313, -6.7621) centre (19.5532, 0.7806) ccw
  arc A402 (18.292, -5.1983) -> (18.5999, -5.2559) centre (19.416, -0.0475) ccw
  arc A403 (18.5999, -5.2559) -> (18.9908, -5.3049) centre (19.5924, 1.0745) ccw
  arc A404 (18.9908, -5.3049) -> (19.476, -5.3351) centre (19.7035, 2.2488) ccw
  arc A405 (18.9154, -3.8105) -> (19.2268, -3.8438) centre (19.6317, 1.4125) ccw
  arc A406 (19.2268, -3.8438) -> (19.6204, -3.862) centre (19.7196, 2.5449) ccw
  arc A407 (19.6204, -3.862) -> (20.1064, -3.854) centre (19.7383, 3.7244) ccw
  arc A408 (19.428, -2.3781) -> (19.741, -2.3869) centre (19.7323, 2.885) ccw
  arc A409 (19.741, -2.3869) -> (20.1348, -2.3742) centre (19.731, 4.0208) ccw
  arc A410 (20.1348, -2.3742) -> (20.6187, -2.3281) centre (19.6571, 5.1981) ccw
  arc A411 (19.8266, -0.91) -> (20.1393, -0.8942) centre (19.717, 4.3608) ccw
  arc A412 (20.1393, -0.8942) -> (20.5309, -0.8506) centre (19.6266, 5.493) ccw
  arc A413 (20.5309, -0.8506) -> (21.0097, -0.7666) centre (19.4606, 6.6609) ccw
  arc A414 (20.1087, 0.585) -> (20.4193, 0.6252) centre (19.586, 5.8309) ccw
  arc A415 (20.4193, 0.6252) -> (20.8062, 0.6994) centre (19.407, 6.9525) ccw
  arc A416 (20.8062, 0.6994) -> (21.277, 0.8207) centre (19.1499, 8.1037) ccw
  arc A417 (20.2728, 2.0974) -> (20.5792, 2.1619) centre (19.34, 7.2862) ccw
  arc A418 (20.5792, 2.1619) -> (20.9591, 2.2662) centre (19.0736, 8.3903) ccw
  arc A419 (20.9591, 2.2662) -> (21.4189, 2.4241) centre (18.7269, 9.5178) ccw
  arc A420 (20.3176, 3.6181) -> (20.618, 3.7064) centre (18.9806, 8.7176) ccw
  arc A421 (20.618, 3.7064) -> (20.9886, 3.8402) centre (18.6284, 9.7974) ccw
  arc A422 (20.9886, 3.8402) -> (21.4346, 4.0336) centre (18.1944, 10.8943) ccw
  arc A423 (20.243, 5.1375) -> (20.5356, 5.2492) centre (18.51, 10.1165) ccw
  arc A424 (20.5356, 5.2492) -> (20.8945, 5.4117) centre (18.0742, 11.1654) ccw
  arc A425 (20.8945, 5.4117) -> (21.3239, 5.6395) centre (17.5554, 12.2248) ccw
  arc A426 (20.0494, 6.6465) -> (20.3323, 6.7808) centre (17.9312, 11.4741) ccw
  arc A427 (20.3323, 6.7808) -> (20.6774, 6.9709) centre (17.4144, 12.4856) ccw
  arc A428 (20.6774, 6.9709) -> (21.0876, 7.2317) centre (16.814, 13.501) ccw
  arc A429 (19.738, 8.1356) -> (20.0095, 8.2917) centre (17.2475, 12.7822) ccw
  arc A430 (20.0095, 8.2917) -> (20.3386, 8.5083) centre (16.653, 13.7499) ccw
  arc A431 (20.3386, 8.5083) -> (20.7271, 8.8005) centre (15.9748, 14.7151) ccw
  arc A432 (19.3108, 9.5957) -> (19.5692, 9.7726) centre (16.4634, 14.0325) ccw
  arc A433 (19.5692, 9.7726) -> (19.8803, 10.0143) centre (15.7947, 14.9507) ccw
  arc A434 (19.8803, 10.0143) -> (20.2447, 10.3361) centre (15.043, 15.8597) ccw
  arc A435 (18.7703, 11.0178) -> (19.014, 11.2144) centre (15.5835, 15.2175) ccw
  arc A436 (19.014, 11.2144) -> (19.3052, 11.4798) centre (14.8449, 16.0804) ccw
  arc A437 (19.3052, 11.4798) -> (19.6432, 11.8292) centre (14.0242, 16.9276) ccw
  arc A438 (18.1199, 12.393) -> (18.3474, 12.6082) centre (14.6135, 16.3298) ccw
  arc A439 (18.3474, 12.6082) -> (18.6169, 12.8956) centre (13.8094, 17.132) ccw
  arc A440 (18.6169, 12.8956) -> (18.9264, 13.2704) centre (12.9247, 17.9123) ccw
  arc A441 (17.3636, 13.713) -> (17.5735, 13.9454) centre (13.5591, 17.3626) ccw
  arc A442 (17.5735, 13.9454) -> (17.8196, 14.2531) centre (12.6946, 18.0992) ccw
  arc A443 (17.8196, 14.2531) -> (18.0988, 14.651) centre (11.7514, 18.8076) ccw
  arc A444 (16.506, 14.9696) -> (16.6971, 15.2177) centre (12.4269, 18.3094) ccw
  arc A445 (16.6971, 15.2177) -> (16.9183, 15.5438) centre (11.5073, 18.976) ccw
  arc A446 (16.9183, 15.5438) -> (17.1654, 15.9624) centre (10.5114, 19.6082) ccw
  arc A447 (15.5525, 16.1551) -> (15.7236, 16.4174) centre (11.224, 19.1645) ccw
  arc A448 (15.7236, 16.4174) -> (15.9185, 16.7598) centre (10.2549, 19.7569) ccw
  arc A449 (15.9185, 16.7598) -> (16.132, 17.1965) centre (9.2125, 20.309) ccw
  arc A450 (14.509, 17.2621) -> (14.6589, 17.537) centre (9.9577, 19.9226) ccw
  arc A451 (14.6589, 17.537) -> (14.8264, 17.8936) centre (8.9451, 20.4371) ccw
  arc A452 (14.8264, 17.8936) -> (15.005, 18.3458) centre (7.8625, 20.9058) ccw
  arc A453 (13.3818, 18.2837) -> (13.5097, 18.5696) centre (8.6357, 20.579) ccw
  arc A454 (13.5097, 18.5696) -> (13.6486, 18.9383) centre (7.5859, 21.0125) ccw
  arc A455 (13.6486, 18.9383) -> (13.7912, 19.403) centre (6.47, 21.3947) ccw
  arc A456 (12.1779, 19.2138) -> (12.283, 19.5089) centre (7.2664, 21.1297) ccw
  arc A457 (12.283, 19.5089) -> (12.3926, 19.8873) centre (6.1858, 21.4794) ccw
  arc A458 (12.3926, 19.8873) -> (12.4983, 20.3618) centre (5.0433, 21.773) ccw
  arc A459 (10.9048, 20.0466) -> (10.9864, 20.349) centre (5.8581, 21.5712) ccw
  arc A460 (10.9864, 20.349) -> (11.0659, 20.7348) centre (4.7534, 21.8351) ccw
  arc A461 (11.0659, 20.7348) -> (11.1341, 21.2162) centre (3.5914, 22.0381) ccw
  arc A462 (9.5702, 20.7769) -> (9.6279, 21.0848) centre (4.4195, 21.9009) ccw
  arc A463 (9.6279, 21.0848) -> (9.6769, 21.4757) centre (3.2975, 22.0773) ccw
  arc A464 (9.6769, 21.4757) -> (9.707, 21.9609) centre (2.1231, 22.1885) ccw
  arc A465 (8.1825, 21.4003) -> (8.2158, 21.7117) centre (2.9594, 22.1166) ccw
  arc A466 (8.2158, 21.7117) -> (8.234, 22.1053) centre (1.827, 22.2045) ccw
  arc A467 (8.234, 22.1053) -> (8.226, 22.5913) centre (0.6476, 22.2232) ccw
  arc A468 (6.7501, 21.9129) -> (6.7589, 22.2259) centre (1.487, 22.2172) ccw
  arc A469 (6.7589, 22.2259) -> (6.7462, 22.6197) centre (0.3512, 22.2159) ccw
  arc A470 (6.7462, 22.6197) -> (6.7, 23.1036) centre (-0.8261, 22.142) ccw
  arc A471 (5.2819, 22.3115) -> (5.2661, 22.6242) centre (0.0111, 22.2019) ccw
  arc A472 (5.2661, 22.6242) -> (5.2225, 23.0158) centre (-1.121, 22.1115) ccw
  arc A473 (5.2225, 23.0158) -> (5.1386, 23.4946) centre (-2.2889, 21.9455) ccw
  arc A474 (3.787, 22.5936) -> (3.7467, 22.9042) centre (-1.4589, 22.0709) ccw
  arc A475 (3.7467, 22.9042) -> (3.6725, 23.2911) centre (-2.5805, 21.8919) ccw
  arc A476 (3.6725, 23.2911) -> (3.5513, 23.7619) centre (-3.7318, 21.6348) ccw
  arc A477 (2.2746, 22.7577) -> (2.21, 23.0641) centre (-2.9142, 21.8249) ccw
  arc A478 (2.21, 23.0641) -> (2.1057, 23.444) centre (-4.0183, 21.5585) ccw
  arc A479 (2.1057, 23.444) -> (1.9479, 23.9038) centre (-5.1458, 21.2118) ccw
  arc A480 (1.1332, 22.8025) -> (0.7539, 22.8025) centre (0.9435, 3.4284) ccw
  arc A481 (-0.3875, 22.7577) -> (-0.7656, 22.7279) centre (0.9435, 3.4284) ccw
  arc A482 (-1.9, 22.5936) -> (-2.2745, 22.5343) centre (0.9435, 3.4284) ccw
  arc A483 (-3.3949, 22.3115) -> (-3.7636, 22.2229) centre (0.9435, 3.4284) ccw
  arc A484 (-4.863, 21.9129) -> (-5.2237, 21.7957) centre (0.9435, 3.4284) ccw
  arc A485 (-6.2954, 21.4003) -> (-6.6458, 21.2552) centre (0.9435, 3.4284) ccw
  arc A486 (-7.6832, 20.7769) -> (-8.0211, 20.6048) centre (0.9435, 3.4284) ccw
  arc A487 (-9.0177, 20.0466) -> (-9.3411, 19.8485) centre (0.9435, 3.4284) ccw
  arc A488 (-10.2909, 19.2138) -> (-10.5977, 18.9909) centre (0.9435, 3.4284) ccw
  arc A489 (-11.4947, 18.2837) -> (-11.7831, 18.0374) centre (0.9435, 3.4284) ccw
  arc A490 (-12.6219, 17.2621) -> (-12.8901, 16.9939) centre (0.9435, 3.4284) ccw
  arc A491 (-13.6655, 16.1551) -> (-13.9118, 15.8667) centre (0.9435, 3.4284) ccw
  arc A492 (-14.619, 14.9696) -> (-14.8419, 14.6628) centre (0.9435, 3.4284) ccw
  arc A493 (-15.4765, 13.713) -> (-15.6747, 13.3897) centre (0.9435, 3.4284) ccw
  arc A494 (-16.2328, 12.393) -> (-16.405, 12.0551) centre (0.9435, 3.4284) ccw
  arc A495 (-16.8832, 11.0178) -> (-17.0283, 10.6674) centre (0.9435, 3.4284) ccw
  arc A496 (-17.4237, 9.5957) -> (-17.5409, 9.235) centre (0.9435, 3.4284) ccw
  arc A497 (-17.851, 8.1356) -> (-17.9395, 7.7668) centre (0.9435, 3.4284) ccw
  arc A498 (-18.1624, 6.6465) -> (-18.2217, 6.2719) centre (0.9435, 3.4284) ccw
  arc A499 (-18.3559, 5.1375) -> (-18.3857, 4.7595) centre (0.9435, 3.4284) ccw
  arc A500 (-18.4305, 3.6181) -> (-18.4305, 3.2388) centre (0.9435, 3.4284) ccw
  arc A501 (-18.3857, 2.0974) -> (-18.3559, 1.7193) centre (0.9435, 3.4284) ccw
  arc A502 (-18.2217, 0.585) -> (-18.1624, 0.2104) centre (0.9435, 3.4284) ccw
  arc A503 (-17.9395, -0.91) -> (-17.851, -1.2787) centre (0.9435, 3.4284) ccw
  arc A504 (-17.5409, -2.3781) -> (-17.4237, -2.7388) centre (0.9435, 3.4284) ccw
  arc A505 (-17.0283, -3.8105) -> (-16.8832, -4.1609) centre (0.9435, 3.4284) ccw
  arc A506 (-16.405, -5.1983) -> (-16.2328, -5.5362) centre (0.9435, 3.4284) ccw
  arc A507 (-15.6747, -6.5328) -> (-15.4765, -6.8562) centre (0.9435, 3.4284) ccw
  arc A508 (-14.8419, -7.8059) -> (-14.619, -8.1128) centre (0.9435, 3.4284) ccw
  arc A509 (-13.9118, -9.0098) -> (-13.6655, -9.2982) centre (0.9435, 3.4284) ccw
  arc A510 (-12.8901, -10.137) -> (-12.6219, -10.4052) centre (0.9435, 3.4284) ccw
  arc A511 (-11.7831, -11.1806) -> (-11.4947, -11.4269) centre (0.9435, 3.4284) ccw
  arc A512 (-10.5977, -12.1341) -> (-10.2909, -12.357) centre (0.9435, 3.4284) ccw
  arc A513 (-9.3411, -12.9916) -> (-9.0177, -13.1898) centre (0.9435, 3.4284) ccw
  arc A514 (-8.0211, -13.7479) -> (-7.6832, -13.9201) centre (0.9435, 3.4284) ccw
  arc A515 (-6.6458, -14.3983) -> (-6.2954, -14.5434) centre (0.9435, 3.4284) ccw
  arc A516 (-5.2237, -14.9388) -> (-4.863, -15.056) centre (0.9435, 3.4284) ccw
  arc A517 (-3.7636, -15.3661) -> (-3.3949, -15.4546) centre (0.9435, 3.4284) ccw
  arc A518 (-2.2745, -15.6774) -> (-1.9, -15.7368) centre (0.9435, 3.4284) ccw
  arc A519 (-0.7656, -15.871) -> (-0.3875, -15.9008) centre (0.9435, 3.4284) ccw
  arc A520 (0.7539, -15.9456) -> (1.1332, -15.9456) centre (0.9435, 3.4284) ccw
  arc A521 (2.2746, -15.9008) -> (2.6526, -15.871) centre (0.9435, 3.4284) ccw
  arc A522 (3.787, -15.7368) -> (4.1616, -15.6774) centre (0.9435, 3.4284) ccw
  arc A523 (5.2819, -15.4546) -> (5.6507, -15.3661) centre (0.9435, 3.4284) ccw
  arc A524 (6.7501, -15.056) -> (7.1108, -14.9388) centre (0.9435, 3.4284) ccw
  arc A525 (8.1825, -14.5434) -> (8.5329, -14.3983) centre (0.9435, 3.4284) ccw
  arc A526 (9.5702, -13.9201) -> (9.9081, -13.7479) centre (0.9435, 3.4284) ccw
  arc A527 (10.9048, -13.1898) -> (11.2281, -12.9916) centre (0.9435, 3.4284) ccw
  arc A528 (12.1779, -12.357) -> (12.4847, -12.1341) centre (0.9435, 3.4284) ccw
  arc A529 (13.3818, -11.4269) -> (13.6702, -11.1806) centre (0.9435, 3.4284) ccw
  arc A530 (14.509, -10.4052) -> (14.7772, -10.137) centre (0.9435, 3.4284) ccw
  arc A531 (15.5525, -9.2982) -> (15.7988, -9.0098) centre (0.9435, 3.4284) ccw
  arc A532 (16.506, -8.1128) -> (16.7289, -7.8059) centre (0.9435, 3.4284) ccw
  arc A533 (17.3636, -6.8562) -> (17.5617, -6.5328) centre (0.9435, 3.4284) ccw
  arc A534 (18.1199, -5.5362) -> (18.292, -5.1983) centre (0.9435, 3.4284) ccw
  arc A535 (18.7703, -4.1609) -> (18.9154, -3.8105) centre (0.9435, 3.4284) ccw
  arc A536 (19.3108, -2.7388) -> (19.428, -2.3781) centre (0.9435, 3.4284) ccw
  arc A537 (19.738, -1.2787) -> (19.8266, -0.91) centre (0.9435, 3.4284) ccw
  arc A538 (20.0494, 0.2104) -> (20.1087, 0.585) centre (0.9435, 3.4284) ccw
  arc A539 (20.243, 1.7193) -> (20.2728, 2.0974) centre (0.9435, 3.4284) ccw
  arc A540 (20.3176, 3.2388) -> (20.3176, 3.6181) centre (0.9435, 3.4284) ccw
  arc A541 (20.2728, 4.7595) -> (20.243, 5.1375) centre (0.9435, 3.4284) ccw
  arc A542 (20.1087, 6.2719) -> (20.0494, 6.6465) centre (0.9435, 3.4284) ccw
  arc A543 (19.8266, 7.7668) -> (19.738, 8.1356) centre (0.9435, 3.4284) ccw
  arc A544 (19.428, 9.235) -> (19.3108, 9.5957) centre (0.9435, 3.4284) ccw
  arc A545 (18.9154, 10.6674) -> (18.7703, 11.0178) centre (0.9435, 3.4284) ccw
  arc A546 (18.292, 12.0551) -> (18.1199, 12.393) centre (0.9435, 3.4284) ccw
  arc A547 (17.5617, 13.3897) -> (17.3636, 13.713) centre (0.9435, 3.4284) ccw
  arc A548 (16.7289, 14.6628) -> (16.506, 14.9696) centre (0.9435, 3.4284) ccw
  arc A549 (15.7988, 15.8667) -> (15.5525, 16.1551) centre (0.9435, 3.4284) ccw
  arc A550 (14.7772, 16.9939) -> (14.509, 17.2621) centre (0.9435, 3.4284) ccw
  arc A551 (13.6702, 18.0374) -> (13.3818, 18.2837) centre (0.9435, 3.4284) ccw
  arc A552 (12.4847, 18.9909) -> (12.1779, 19.2138) centre (0.9435, 3.4284) ccw
  arc A553 (11.2281, 19.8485) -> (10.9048, 20.0466) centre (0.9435, 3.4284) ccw
  arc A554 (9.9081, 20.6048) -> (9.5702, 20.7769) centre (0.9435, 3.4284) ccw
  arc A555 (8.5329, 21.2552) -> (8.1825, 21.4003) centre (0.9435, 3.4284) ccw
  arc A556 (7.1108, 21.7957) -> (6.7501, 21.9129) centre (0.9435, 3.4284) ccw
  arc A557 (5.6507, 22.2229) -> (5.2819, 22.3115) centre (0.9435, 3.4284) ccw
  arc A558 (4.1616, 22.5343) -> (3.787, 22.5936) centre (0.9435, 3.4284) ccw
  arc A559 (2.6526, 22.7279) -> (2.2746, 22.7577) centre (0.9435, 3.4284) ccw
  arc A560 (0.3383, 23.9195) -> (-0.0608, 23.9038) centre (0.9435, 3.4284) ccw
  arc A561 (-1.2675, 23.8088) -> (-1.6642, 23.7619) centre (0.9435, 3.4284) ccw
  arc A562 (-2.8597, 23.5725) -> (-3.2515, 23.4946) centre (0.9435, 3.4284) ccw
  arc A563 (-4.4285, 23.212) -> (-4.813, 23.1036) centre (0.9435, 3.4284) ccw
  arc A564 (-5.9641, 22.7296) -> (-6.3389, 22.5913) centre (0.9435, 3.4284) ccw
  arc A565 (-7.4572, 22.1281) -> (-7.82, 21.9609) centre (0.9435, 3.4284) ccw
  arc A566 (-8.8985, 21.4113) -> (-9.247, 21.2162) centre (0.9435, 3.4284) ccw
  arc A567 (-10.279, 20.5837) -> (-10.6112, 20.3618) centre (0.9435, 3.4284) ccw
  arc A568 (-11.5904, 19.6503) -> (-11.9041, 19.403) centre (0.9435, 3.4284) ccw
  arc A569 (-12.8246, 18.6169) -> (-13.1179, 18.3458) centre (0.9435, 3.4284) ccw
  arc A570 (-13.9738, 17.4899) -> (-14.2449, 17.1965) centre (0.9435, 3.4284) ccw
  arc A571 (-15.0311, 16.2761) -> (-15.2784, 15.9624) centre (0.9435, 3.4284) ccw
  arc A572 (-15.9898, 14.9832) -> (-16.2118, 14.651) centre (0.9435, 3.4284) ccw
  arc A573 (-16.8442, 13.619) -> (-17.0394, 13.2704) centre (0.9435, 3.4284) ccw
  arc A574 (-17.5889, 12.1919) -> (-17.7561, 11.8292) centre (0.9435, 3.4284) ccw
  arc A575 (-18.2193, 10.7109) -> (-18.3576, 10.3361) centre (0.9435, 3.4284) ccw
  arc A576 (-18.7317, 9.1849) -> (-18.8401, 8.8005) centre (0.9435, 3.4284) ccw
  arc A577 (-19.1226, 7.6235) -> (-19.2006, 7.2317) centre (0.9435, 3.4284) ccw
  arc A578 (-19.3899, 6.0362) -> (-19.4369, 5.6395) centre (0.9435, 3.4284) ccw
  arc A579 (-19.5319, 4.4328) -> (-19.5475, 4.0336) centre (0.9435, 3.4284) ccw
  arc A580 (-19.5475, 2.8232) -> (-19.5319, 2.4241) centre (0.9435, 3.4284) ccw
  arc A581 (-19.4369, 1.2174) -> (-19.3899, 0.8207) centre (0.9435, 3.4284) ccw
  arc A582 (-19.2006, -0.3748) -> (-19.1226, -0.7666) centre (0.9435, 3.4284) ccw
  arc A583 (-18.8401, -1.9436) -> (-18.7317, -2.3281) centre (0.9435, 3.4284) ccw
  arc A584 (-18.3576, -3.4792) -> (-18.2193, -3.854) centre (0.9435, 3.4284) ccw
  arc A585 (-17.7561, -4.9723) -> (-17.5889, -5.3351) centre (0.9435, 3.4284) ccw
  arc A586 (-17.0394, -6.4136) -> (-16.8442, -6.7621) centre (0.9435, 3.4284) ccw
  arc A587 (-16.2118, -7.7941) -> (-15.9898, -8.1263) centre (0.9435, 3.4284) ccw
  arc A588 (-15.2784, -9.1055) -> (-15.0311, -9.4192) centre (0.9435, 3.4284) ccw
  arc A589 (-14.2449, -10.3397) -> (-13.9738, -10.633) centre (0.9435, 3.4284) ccw
  arc A590 (-13.1179, -11.4889) -> (-12.8246, -11.76) centre (0.9435, 3.4284) ccw
  arc A591 (-11.9041, -12.5461) -> (-11.5904, -12.7935) centre (0.9435, 3.4284) ccw
  arc A592 (-10.6112, -13.5049) -> (-10.279, -13.7268) centre (0.9435, 3.4284) ccw
  arc A593 (-9.247, -14.3593) -> (-8.8985, -14.5545) centre (0.9435, 3.4284) ccw
  arc A594 (-7.82, -15.104) -> (-7.4572, -15.2712) centre (0.9435, 3.4284) ccw
  arc A595 (-6.3389, -15.7344) -> (-5.9641, -15.8727) centre (0.9435, 3.4284) ccw
  arc A596 (-4.813, -16.2467) -> (-4.4285, -16.3552) centre (0.9435, 3.4284) ccw
  arc A597 (-3.2515, -16.6377) -> (-2.8597, -16.7157) centre (0.9435, 3.4284) ccw
  arc A598 (-1.6642, -16.905) -> (-1.2675, -16.952) centre (0.9435, 3.4284) ccw
  arc A599 (-0.0608, -17.0469) -> (0.3383, -17.0626) centre (0.9435, 3.4284) ccw
  arc A600 (1.5487, -17.0626) -> (1.9479, -17.0469) centre (0.9435, 3.4284) ccw
  arc A601 (3.1546, -16.952) -> (3.5513, -16.905) centre (0.9435, 3.4284) ccw
  arc A602 (4.7468, -16.7157) -> (5.1386, -16.6377) centre (0.9435, 3.4284) ccw
  arc A603 (6.3156, -16.3552) -> (6.7, -16.2467) centre (0.9435, 3.4284) ccw
  arc A604 (7.8512, -15.8727) -> (8.226, -15.7344) centre (0.9435, 3.4284) ccw